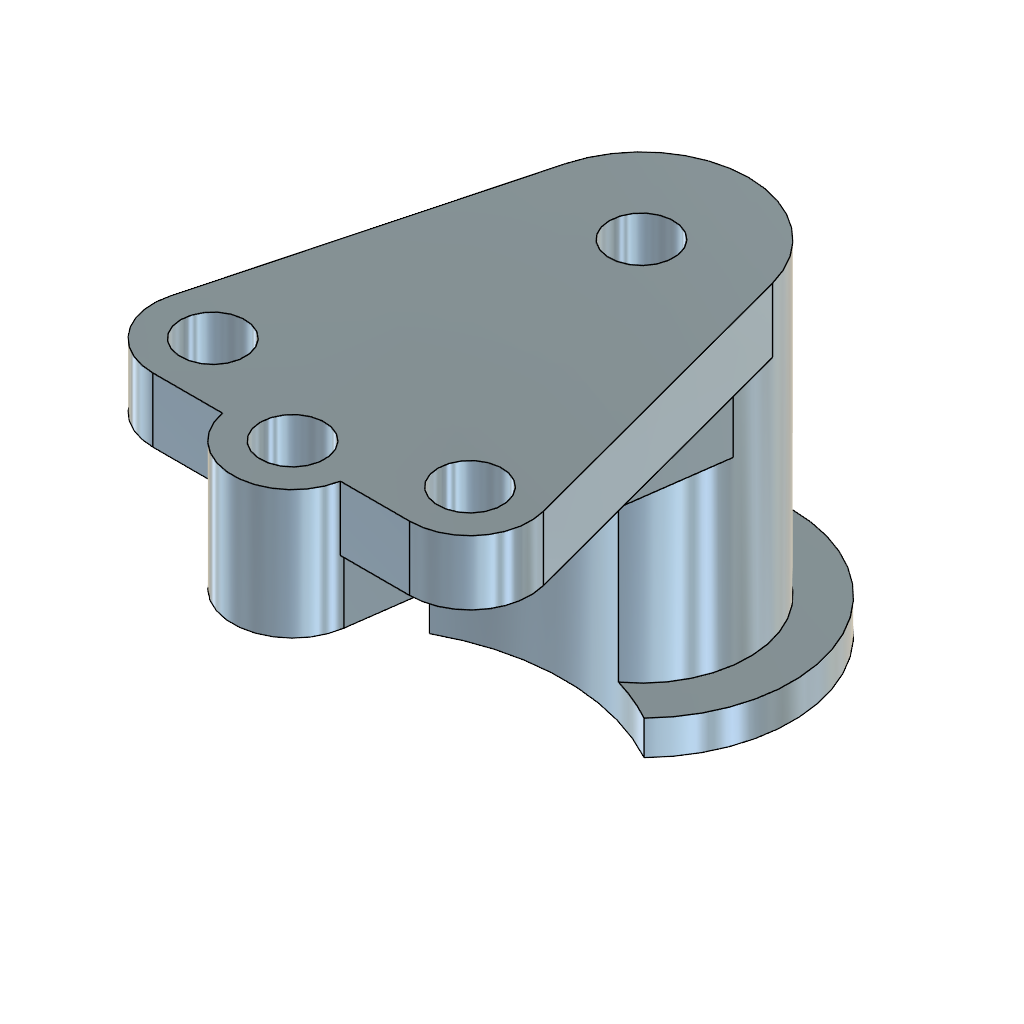
8th 3d design triangular mounting bracket (Autodesk Fusion 360 design; units mm, degrees)
part number: 2026-01-20-20-01-35-274
Autodesk Fusion 360 part; units mm, degrees
note: some values were not read from the file. Set by a fixed rule: which sketch regions a step uses.
sketch "Sketch1" plane through (0, 0, 0) normal (0, 0, 1) x (1, 0, 0)
  circle A0 centre (0, 0) radius 7.5
  circle A1 centre (30, -70) radius 7.5
  circle A2 centre (-30, -70) radius 7.5
  line L0 (24.1601, 6.4258) -> (43.5296, -66.4016)
  line L1 (-24.1601, 6.4258) -> (-43.5296, -66.4016)
  line L2 (29.8941, -83.9996) -> (-29.9999, -84)
  arc A3 (24.1601, 6.4258) -> (-24.1601, 6.4258) centre (0, 0) ccw
  arc A4 (29.8941, -83.9996) -> (43.5296, -66.4016) centre (30, -70) ccw
  arc A5 (-43.5296, -66.4016) -> (-29.9999, -84) centre (-30, -70) ccw
  dimension "d10" = 15
  dimension "d11" = 15
  dimension "d12" = 28
  dimension "d13" = 15
  dimension "d14" = 28
  dimension "d15" = 70
  dimension "d16" = 60
  dimension "d17" = 30
  dimension "d19" = 50
  constraint coincident A0.centre A3.centre
  constraint concentric A1 A4
  constraint concentric A2 A5
  constraint horizontal A1.centre A2.centre
  constraint concentric A0 A3
  constraint tangent L0 A4
  constraint tangent L1 A5
  constraint tangent L2 A5
  constraint tangent L0 A3
  constraint tangent L1 A3
  measures "d10" diameter of A0
  measures "d11" diameter of A1
  measures "d12" diameter of A4
  measures "d13" diameter of A2
  measures "d14" diameter of A5
  measures "d15" vertical distance of A0.centre A1.centre
  measures "d16" distance of A1.centre A2.centre
  measures "d17" horizontal distance of A0.centre A1.centre
  measures "d19" diameter of A3
extrude "Extrude1" add sketch "Sketch1" along normal blind 15 makes body 1
sketch "Sketch2" plane through (0, 0, 0) normal (0, 0, -1) x (1, 0, 0)
  circle A0 centre (30, 70) radius 7.5
  circle A1 centre (0, 0) radius 7.5
  circle A2 centre (-30, 70) radius 7.5
  arc A3 (-24.1601, -6.4258) -> (24.1601, -6.4258) centre (0, 0) ccw
  line L0 (24.1601, -6.4258) -> (43.5296, 66.4016)
  arc A4 (43.5296, 66.4016) -> (29.8941, 83.9996) centre (30, 70) ccw
  line L1 (29.8941, 83.9996) -> (-29.9999, 84)
  arc A5 (-29.9999, 84) -> (-43.5296, 66.4016) centre (-30, 70) ccw
  line L2 (-43.5296, 66.4016) -> (-24.1601, -6.4258)
  line L3 (24.7707, 3.3785) -> (13.8716, 83.2887)
  line L4 (-24.7707, 3.3785) -> (-13.8716, 83.2887)
  arc A6 (13.8716, 83.2887) -> (-13.8716, 83.2887) centre (0, 81.3967) ccw
  arc A7 (-24.7707, 3.3785) -> (24.7707, 3.3785) centre (0, 0) ccw
  dimension "d22" = 28
  constraint coincident A1.centre A3.centre
  constraint coincident A3.end A7
  constraint tangent L3 A6
  constraint tangent L4 A6
  constraint tangent L3 A7
  constraint tangent L4 A7
  constraint vertical A1.centre A6.centre
  measures "d22" diameter of A6
extrude "Extrude2" add sketch "Sketch2" along normal mid plane 30 contours A3 L1 L3 L4 A6 A7 | L1 A6 bodies 1
sketch "Sketch3" plane through (0, 0, -15) normal (0, 0, -1) x (1, 0, 0)
  circle A0 centre (0, 0) radius 7.5
  arc A1 (-24.7707, 3.3785) -> (24.7707, 3.3785) centre (0, 0) ccw
  line L0 (24.7707, 3.3785) -> (13.8716, 83.2887)
  arc A2 (13.8716, 83.2887) -> (-13.8716, 83.2887) centre (0, 81.3967) ccw
  line L1 (-13.8716, 83.2887) -> (-24.7707, 3.3785)
  circle A3 centre (0, 81.3967) radius 7.5
  dimension "d25" = 15
  constraint concentric A2 A3
  measures "d25" diameter of A3
extrude "Extrude3" cut sketch "Sketch3" against normal blind 295 contours A3 bodies 1
sketch "Sketch4" plane through (0, 0, -15) normal (0, 0, -1) x (1, 0, 0)
  circle A0 centre (0, 81.3967) radius 7.5
  circle A1 centre (0, 0) radius 7.5
  arc A2 (-24.7707, 3.3785) -> (24.7707, 3.3785) centre (0, 0) ccw
  line L0 (24.7707, 3.3785) -> (13.8716, 83.2887)
  arc A3 (13.8716, 83.2887) -> (-13.8716, 83.2887) centre (0, 81.3967) ccw
  line L1 (-13.8716, 83.2887) -> (-24.7707, 3.3785)
  circle A4 centre (0, 0) radius 25
  constraint coincident A1.centre A2.centre
  constraint coincident A2.start A4
extrude "Extrude4" add sketch "Sketch4" along normal blind 42 contours A2 A4 bodies 1
sketch "Sketch5" plane through (0, 0, -57) normal (0, 0, -1) x (1, 0, 0)
  circle A0 centre (0, 0) radius 7.5
  circle A1 centre (0, 0) radius 25
  circle A2 centre (0, 0) radius 35
  dimension "d30" = 70
  constraint coincident A0.centre A1.centre
  measures "d30" diameter of A2
extrude "Extrude5" add sketch "Sketch5" along normal blind 8 separate body contours A2 makes body 2
extrude "Extrude6" add 1 faces at (-19.0895, -1.0145, -57) along direction (0, 0, -1) blind 8 on bodies 1 bodies 1 2
sketch "Sketch6" plane through (0, 0, -65) normal (0, 0, -1) x (1, 0, 0)
  circle A0 centre (0, 0) radius 7.5
  circle A1 centre (0, 0) radius 35
  circle A2 centre (0, 70) radius 52
  dimension "d36" = 104
  dimension "d37" = 70
  measures "d36" diameter of A2
  measures "d37" distance of A0.centre A2.centre
extrude "Extrude7" cut sketch "Sketch6" against normal up to surface (50 mm away) contours A1 A2 picked at (0.8456, 23.7254) bodies 1
